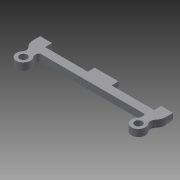
# Autodesk Inventor part: HDMIPluginModuleHolder03
Saved by Autodesk Inventor 2015 (Build 190159000, 159)
## iProperties
Created: 2015-10-14
Part Number: HDMIPluginModuleHolder03
Material: Generic
Document SubType Name: Modeling
Designer: -
Density: 1 g/cm^3
Appearance: Default
Author: -
Autodesk Inventor part; units mm, degrees
ref_plane "YZ Plane" through (0, 0, 0) normal (1, 0, 0) x (0, 1, 0)
ref_plane "XZ Plane" through (0, 0, 0) normal (0, 1, 0) x (-1, 0, 0)
ref_plane "XY Plane" through (0, 0, 0) normal (0, 0, 1) x (1, 0, 0)
sketch "Sketch1" plane through (0, 0, 0) normal (0, 1, 0) x (-1, 0, 0)
  circle A0 centre (0, 0) radius 1.65
  line L0 (0, 0) -> (22.8671, 0) construction
  circle A1 centre (-49.53, 0) radius 1.65
  circle A2 centre (-49.53, 0) radius 3
  line L1 (-24.765, 0) -> (-24.765, 33.4897) construction
  line L2 (0, 0) -> (0, -6.322) construction
  line L3 (-49.53, 0) -> (-44.53, 0) construction
  circle A3 centre (0, 0) radius 3
  dimension "d0" = 3.3
  dimension "d2" = 49.53
  dimension "d3" = 3.3
  dimension "d4" = 6
  dimension "d11" = 6
  constraints: 8 end point, 4 centre point, 3 coincident, 2 horizontal, 2 vertical, 1 point on line
  measures "d0" diameter of A0
  measures "d2" distance of L0.start A1.centre
  measures "d3" diameter of A1
  measures "d4" diameter of A2
  measures "d11" diameter of A3
extrude "Extrusion1" add sketch "Sketch1" along normal blind 3
sketch "Sketch2" plane through (49.53, 0, 0) normal (0, -1, 0) x (1, 0, 0)
  line L0 (1.75, -2.2) -> (1.75, -6.339)
  line L1 (-0.25, -8.339) -> (-49.28, -8.339)
  line L2 (-51.28, -6.339) -> (-51.28, -2.2)
  line L3 (-47.78, -2.2) -> (-47.78, -3.839)
  line L4 (-46.78, -4.839) -> (-2.75, -4.839)
  line L5 (-1.75, -3.839) -> (-1.75, -2.2)
  line L6 (0, 0) -> (0, -7.7115) construction
  line L7 (1.75, -2.2) -> (-1.75, -2.2)
  line L8 (-49.53, 0) -> (-49.53, -7.2415) construction
  line L9 (-47.78, -2.2) -> (-51.28, -2.2)
  arc A0 (-47.78, -3.839) -> (-46.78, -4.839) centre (-46.78, -3.839) ccw
  arc A1 (-2.75, -4.839) -> (-1.75, -3.839) centre (-2.75, -3.839) ccw
  arc A2 (-51.28, -6.339) -> (-49.28, -8.339) centre (-49.28, -6.339) ccw
  arc A3 (-0.25, -8.339) -> (1.75, -6.339) centre (-0.25, -6.339) ccw
  point P0 (1.75, -8.339)
  point P1 (0, -2.2)
  point P2 (-49.53, -2.2)
  dimension "d14" = 6.139
  dimension "d15" = 2.2
  dimension "d16" = 3.5
  dimension "d17" = 3.5
  dimension "d18" = 2.2
  dimension "d19" = 1
  dimension "d20" = 2
  constraints: 20 end point, 8 point on circle, 8 tangent, 4 centre point, 4 perpendicular, 4 point on line, 3 vertical, 2 equal radius, 2 horizontal, 2 midpoint, 2 other
  measures "d14" distance of L0.start point (1.75, -8.339)
  measures "d15" distance from line of L6.start L7
  measures "d16" distance between parallel lines of L0 L5
  measures "d17" distance between parallel lines of L4 L1
  measures "d18" distance from line of L8.start L9
  measures "d19" radius of A0
  measures "d20" radius of A2
extrude "Extrusion2" add sketch "Sketch2" against normal blind 3
sketch "Sketch3" plane through (49.28, 0, -8.339) normal (0, 0, -1) x (-1, 0, 0)
  arc A0 (21.6693, 0.5715) -> (22.8123, 0.5715) centre (22.2408, 0.5715) ccw
  line L0 (49.03, 0) -> (0, 0) construction
  line L1 (0, 3) -> (49.03, 3) projected
  line L2 (-2, 0) -> (-2, 3) projected
  line L3 (22.8123, 0.5715) -> (22.8123, 1.2065)
  line L4 (22.8123, 1.2065) -> (24.8123, 1.2065)
  line L5 (24.8123, 1.2065) -> (24.8123, 3)
  line L6 (21.6693, 0.5715) -> (21.6693, 1.2065)
  line L7 (21.6693, 1.2065) -> (19.6693, 1.2065)
  line L8 (19.6693, 1.2065) -> (19.6693, 3)
  line L9 (22.2408, 0.5715) -> (23.4157, 0.5715) construction
  line L10 (24.8123, 3) -> (19.6693, 3)
  point P0 (49.28, 0)
  point P1 (46.53, 3)
  point P2 (2.5, 3)
  dimension "d23" = 1.143
  dimension "d26" = 24.2408
  dimension "d27" = 2
  dimension "d28" = 2
  dimension "d29" = 0.635
  dimension "d30" = 0.635
  dimension "d31" = 2.4285
  constraints: 16 end point, 3 perpendicular, 2 collinear, 2 horizontal, 2 point on circle, 2 point on line, 2 vertical, 1 centre point, 1 coincident, 1 tangent
  measures "d23" diameter of A0
  measures "d26" distance from line of A0.centre L2
  measures "d27" distance of L3.end L4.end
  measures "d28" distance of L6.end L7.end
  measures "d29" distance of L6.start L6.end
  measures "d30" distance of L3.start L3.end
  measures "d31" distance from line of L9.start L10
extrude "Extrusion3" add sketch "Sketch3" along normal blind 3
pattern_linear "Rectangular Pattern1" count 2 spacing 23.495 along (1, 0, 0) of "Extrusion3"
sketch "Sketch4" plane through (47.9627, 3, -8.339) normal (0, 1, 0) x (1, 0, 0)
  arc A0 (0, -5.143) -> (5.143, 0) centre (0, 0) ccw
  line L0 (5.143, 0) -> (0, 0)
  line L1 (0, 0) -> (0, -5.143)
  point P0 (-47.9627, -8.339)
  constraints: 4 end point, 2 point on circle, 1 centre point, 1 horizontal, 1 perpendicular
extrude "Extrusion4" add sketch "Sketch4" against normal blind 3
pattern_linear "Rectangular Pattern2" count 2 spacing 5.08 along (-1, 0, 0) of "Extrusion3"
pattern_linear "Rectangular Pattern3" count 2 spacing 23.495 along (-1, 0, 0) of "Rectangular Pattern2"
sketch "Sketch6" plane through (0, 0, 0) normal (0, -1, 0) x (1, 0, 0)
  line L0 (1.0357, -8.339) -> (-4.1073, -8.339)
  line L1 (-4.1073, -8.339) -> (-1.6483, -8.339)
  line L2 (-0.2103, -8.339) -> (0.25, -8.339)
  line L3 (0.25, -8.339) -> (1.0357, -8.339)
  line L4 (1.0357, -8.339) -> (1.0357, -3.196)
  arc A0 (1.0357, -3.196) -> (-4.1073, -8.339) centre (1.0357, -8.339) ccw
  line L5 (-0.9643, -8.339) -> (0.25, -8.339) projected
  line L6 (-0.9643, -8.339) -> (-0.9643, -11.339) projected
  line L7 (1.0357, -11.339) -> (-0.9643, -11.339) projected
  line L8 (1.0357, -8.339) -> (1.0357, -11.339) projected
  line L9 (0.25, -8.339) -> (1.0357, -8.339) projected
  line L10 (-4.1073, -8.339) -> (-2.1073, -8.339) projected
  line L11 (-4.1073, -8.339) -> (-4.1073, -11.339) projected
  line L12 (-2.1073, -11.339) -> (-4.1073, -11.339) projected
  line L13 (-2.1073, -8.339) -> (-2.1073, -11.339) projected
  line L14 (0.25, -8.339) -> (21.9592, -8.339) projected
  point P0 (5.143, 0)
  constraints: 10 end point, 5 point on line, 2 point on circle, 1 centre point, 1 coincident, 1 vertical
extrude "Extrusion5" add sketch "Sketch6" against normal blind 3 contours L0 A0 L4
sketch "Sketch7" plane through (53.1057, 3, -11.339) normal (0, 0, -1) x (-1, 0, 0)
  line L0 (3.143, -2.4285) -> (3.143, -1.7935) construction
  line L1 (3.143, -1.7935) -> (5.143, -1.7935) construction
  line L2 (5.143, -1.7935) -> (5.143, 0) construction
  line L3 (5.143, 0) -> (0, 0) construction
  line L4 (0, 0) -> (0, -1.7935) construction
  line L5 (0, -1.7935) -> (2, -1.7935) construction
  line L6 (2, -1.7935) -> (2, -2.4285) construction
  arc A0 (2, -2.4285) -> (3.143, -2.4285) centre (2.5715, -2.4285) ccw construction
  line L7 (0, -1.7935) -> (0, 0)
  line L8 (0, 0) -> (5.143, 0)
  line L9 (5.143, 0) -> (5.143, -1.7935)
  arc A1 (0, -1.7935) -> (5.143, -1.7935) centre (2.5715, -1.7935) ccw
  line L10 (5.143, -1.7935) -> (0, -1.7935) construction
  line L11 (5.143, -1.7935) -> (5.143, 0) construction
  point P0 (53.1057, -3)
  constraints: 8 end point, 3 perpendicular, 2 point on circle, 1 centre point, 1 coincident, 1 midpoint, 1 vertical
extrude "Extrusion6" add sketch "Sketch7" against normal blind 1.2
pattern_linear "Rectangular Pattern4" count 2 spacing 23.495 along (-1, 0, 0) of "Extrusion6"
pattern_linear "Rectangular Pattern5" count 2 spacing 28.575 along (-1, 0, 0) of "Extrusion6"
pattern_linear "Rectangular Pattern6" count 2 spacing 52.07 along (-1, 0, 0) of "Extrusion6"
sketch "Sketch9" plane through (0, 0, 0) normal (0, -1, 0) x (1, 0, 0)
  circle A0 centre (0, 0) radius 1.65 projected
  circle A1 centre (49.53, 0) radius 1.65 projected
  circle A2 centre (49.53, 0) radius 3.5
  arc A3 (1.75, -2.4367) -> (-1.75, -2.4367) centre (0, 0) ccw projected
  circle A4 centre (0, 0) radius 3.5
  point P0 (2.1649, -2.7501)
  constraints: 2 centre point, 2 coincident, 1 other
extrude "Extrusion7" [suppressed]
fillet "Fillet2" radius 2 2 edges at (1.75, 1.5, -2.4367) (47.78, 1.5, -2.4367)
fillet "Fillet3" radius 2 4 edges at (-1.75, 1.5, -2.4367) (51.28, 1.5, -2.4367) (51.28, 1.5, -4.4088) (-1.75, 1.5, -4.0158)
body "Solid1"
